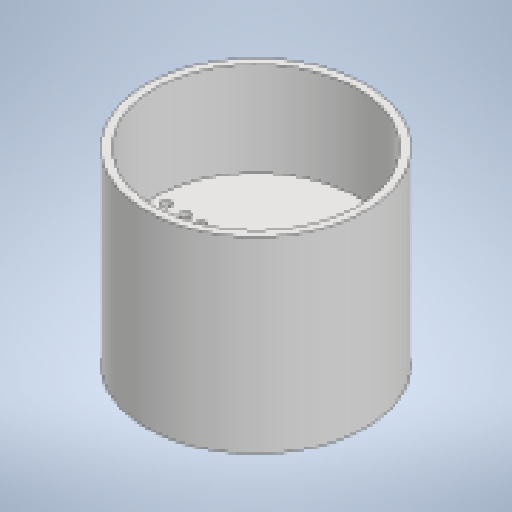
# Autodesk Inventor part: Grundkörper
Saved by Autodesk Inventor 2024 (Build 280153000, 153)
## iProperties
Created: 2024-02-13
Part Number: Grundkörper
Material: Generic
Document SubType Name: Modeling
Designer: Daniel Nussbaum
Density: 1 g/cm^3
Appearance: Default
Author: Daniel Nussbaum
Autodesk Inventor part; units mm, degrees
ref_plane "YZ Plane" through (0, 0, 0) normal (1, 0, 0) x (0, 1, 0)
ref_plane "XZ Plane" through (0, 0, 0) normal (0, 1, 0) x (-1, 0, 0)
ref_plane "XY Plane" through (0, 0, 0) normal (0, 0, 1) x (1, 0, 0)
sketch "Sketch1" plane through (0, 0, 0) normal (0, 0, 1) x (1, 0, 0)
  line L0 (0, 0) -> (0, 25)
  line L1 (0, 60) -> (35, 60)
  line L2 (35, 60) -> (35, 0)
  line L3 (35, 0) -> (30, 0)
  line L4 (35, 0) -> (0, 35)
  line L5 (35, 0) -> (30, 0)
  line L6 (30, 0) -> (30, 5)
  line L7 (30, 5) -> (32.5, 5)
  line L8 (35, 5) -> (35, 0)
  line L9 (30, 5) -> (25, 5)
  line L10 (25, 5) -> (25, 10)
  line L11 (25, 10) -> (30, 10)
  line L12 (30, 10) -> (30, 5)
  line L13 (25, 10) -> (20, 10)
  line L14 (20, 10) -> (20, 15)
  line L15 (20, 15) -> (25, 15)
  line L16 (25, 15) -> (25, 10)
  line L17 (20, 15) -> (15, 15)
  line L18 (15, 15) -> (15, 20)
  line L19 (15, 20) -> (20, 20)
  line L20 (20, 20) -> (20, 15)
  line L21 (15, 20) -> (10, 20)
  line L22 (10, 20) -> (10, 25)
  line L23 (10, 25) -> (15, 25)
  line L24 (15, 25) -> (15, 20)
  line L25 (10, 25) -> (0, 25)
  line L26 (0, 25) -> (0, 60)
  line L27 (30, 0) -> (0, 0)
  line L28 (32.5, 60) -> (32.5, 0)
  line L29 (32.5, 5) -> (35, 5)
  line L30 (27.5, 10) -> (32.5, 10)
  line L31 (0, 30) -> (10, 30)
  line L32 (10, 30) -> (32.5, 30)
  point P0 (5, 30)
  point P1 (32.5, 0)
  dimension "d0" = 60
  dimension "d1" = 35
  dimension "d2" = 45
  dimension "d3" = 5
  dimension "d4" = 5
  dimension "d5" = 5
  dimension "d6" = 5
  dimension "d7" = 5
  dimension "d8" = 2.5
  dimension "d9" = 5
  constraints: 66 end point, 14 point on line, 11 parallel, 11 perpendicular, 6 horizontal, 3 midpoint, 2 vertical
  measures "d0" distance of L0.start L1.start
  measures "d1" distance of L1.start L1.end
  measures "d2" angle of L2 L4
  measures "d3" distance of L6.end L8.start
  measures "d4" distance of L10.end L11.end
  measures "d5" distance of L14.end L15.end
  measures "d6" distance of L18.end L19.end
  measures "d7" distance of L22.end L23.end
  measures "d8" distance between parallel lines of L2 L28
  measures "d9" distance between parallel lines of L25 L31
revolve "Revolution1" add sketch "Sketch1" angle 360 about axis through (0, 25, 0) along (0, 1, 0) contours L26 L31 L4 L25 | L4 L31 L32 L28 L30 L11 L16 L15 L20 L19 L24 L23 | L28 L4 L3 | L4 L28 L29 L2 | L28 L1 L2 L29
sketch "Sketch4" plane through (0, 10, 0) normal (0, -1, 0) x (1, 0, 0)
  circle A0 centre (0, 0) radius 32.5 projected
  circle A1 centre (0, 0) radius 25 projected
  line L0 (-32.5, 0) -> (-25, 0)
  point P0 (-28.75, 0)
  constraints: 2 end point, 2 horizontal alignment, 1 horizontal, 1 midpoint, 2 other
sketch "Sketch5" plane through (0, 15, 0) normal (0, -1, 0) x (1, 0, 0)
  circle A0 centre (0, 0) radius 25 projected
  circle A1 centre (0, 0) radius 20 projected
  line L0 (-25, 0) -> (-20, 0)
  point P0 (-22.5, 0)
  constraints: 2 end point, 2 horizontal alignment, 1 horizontal, 1 midpoint, 2 other
sketch "Sketch6" plane through (0, 20, 0) normal (0, -1, 0) x (1, 0, 0)
  circle A0 centre (0, 0) radius 20 projected
  circle A1 centre (0, 0) radius 15 projected
  line L0 (-20, 0) -> (-15, 0)
  point P0 (-17.5, 0)
  constraints: 2 end point, 2 horizontal alignment, 1 horizontal, 1 midpoint, 2 other
sketch "Sketch7" plane through (0, 25, 0) normal (0, -1, 0) x (1, 0, 0)
  circle A0 centre (0, 0) radius 15 projected
  line L0 (-15, 0) -> (-12.5, 0)
  dimension "d19" = 2.5
  constraints: 2 end point, 1 coincident, 1 horizontal, 1 horizontal alignment, 1 other
  measures "d19" distance of L0.start L0.end
hole "Hole2" at (-28.75, 10, 0) direction (0, 1, 0) diameter 3 end through all counterbore diameter 4.5 counterbore depth 3
hole "Hole3" at (-22.5, 15, 0) direction (0, 1, 0) diameter 3 end through all counterbore diameter 4 counterbore depth 3
hole "Hole4" at (-17.5, 20, 0) direction (0, 1, 0) diameter 3 end through all counterbore diameter 4.5 counterbore depth 3
hole "Hole5" at (-12.5, 25, 0) direction (0, 1, 0) diameter 3 end through all counterbore diameter 4.5 counterbore depth 3
sketch "Sketch8" plane through (0, 0, 0) normal (0, 0, 1) x (1, 0, 0)
  line L0 (35, 60) -> (-35, 60) projected
  line L1 (35, 0) -> (-35, 0) projected
  line L2 (32.5, 60) -> (-32.5, 60) projected
  line L3 (0, 60) -> (0, 55)
  circle A0 centre (0, 55) radius 1.5
  point P0 (0, 0)
  dimension "d48" = 5
  dimension "d49" = 3
  constraints: 2 end point, 1 centre point, 1 coincident, 1 midpoint, 1 vertical
  measures "d48" distance of L3.start L3.end
  measures "d49" diameter of A0
extrude "Extrusion1" cut sketch "Sketch8" along normal through all both and the other way through all
sketch "Sketch9" plane through (0, 0, 0) normal (1, 0, 0) x (0, 1, 0)
  line L0 (60, -35) -> (60, 35) projected
  line L1 (0, -35) -> (0, 35) projected
  line L2 (60, 0) -> (55, 0)
  circle A0 centre (55, 0) radius 1.5
  point P0 (0, 0)
  point P1 (55, 34.9678)
  point P2 (55, -34.9678)
  dimension "d52" = 5
  dimension "d53" = 3
  constraints: 2 end point, 1 centre point, 1 coincident, 1 horizontal, 1 midpoint
  measures "d52" distance of L2.start L2.end
  measures "d53" diameter of A0
extrude "Extrusion2" cut sketch "Sketch9" along normal through all both and the other way through all
body "Solid1"
